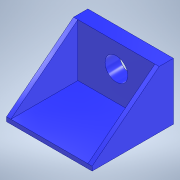
# Autodesk Inventor part: Motor Mount
Saved by Autodesk Inventor 2022 (Build 260153000, 153)
## iProperties
Created: 2022-08-10
Part Number: Motor Mount
Material: Generic
Document SubType Name: Modeling
Designer: Nick
Density: 1 g/cm^3
Appearance: Blue - Wall Paint - Glossy
Author: Nick
Autodesk Inventor part; units mm, degrees
ref_plane "YZ Plane" through (0, 0, 0) normal (1, 0, 0) x (0, 1, 0)
ref_plane "XZ Plane" through (0, 0, 0) normal (0, 1, 0) x (-1, 0, 0)
ref_plane "XY Plane" through (0, 0, 0) normal (0, 0, 1) x (1, 0, 0)
sketch "Sketch14" plane through (0, 0, 0) normal (0, 0, 1) x (1, 0, 0)
  line L0 (0, 0) -> (60, 0)
  line L1 (60, 0) -> (60, 40)
  line L2 (60, 40) -> (0, 40)
  line L3 (0, 40) -> (0, 0)
  circle A0 centre (30, 23.5) radius 8
  point P0 (60, 20)
  point P1 (30, 40)
  dimension "d94" = 16
  dimension "d95" = 60
  dimension "d96" = 40
  dimension "d104" = 23.5
  constraints: 8 end point, 2 midpoint, 2 parallel, 1 centre point, 1 horizontal, 1 perpendicular, 1 vertical alignment
  measures "d94" diameter of A0
  measures "d95" distance of L0.start L0.end
  measures "d96" distance of L2.end L0.start
  measures "d104" distance from line of L0 A0.centre
extrude "Extrusion13" add sketch "Sketch14" along normal blind 10
sketch "Sketch15" plane through (0, 0, 0) normal (0, -1, 0) x (1, 0, 0)
  line L0 (0, 0) -> (60, 0) projected
  line L1 (60, 0) -> (60, 10) projected
  line L2 (0, 10) -> (60, 10) projected
  line L3 (0, 0) -> (0, 10) projected
  line L4 (60, 0) -> (60, 10) projected
  line L5 (60, 10) -> (0, 10)
  line L6 (0, 10) -> (0, 57)
  line L7 (0, 57) -> (60, 57)
  line L8 (60, 57) -> (60, 10)
  line L9 (0, 0) -> (0, 10) projected
  dimension "d99" = 47
  constraints: 8 end point, 2 parallel, 1 collinear, 1 horizontal, 1 perpendicular
  measures "d99" distance of L7.end L1.end
extrude "Extrusion14" add sketch "Sketch15" against normal blind 3 contours L6 L7 L8 L2
sketch "Sketch16" plane through (60, 0, 0) normal (1, 0, 0) x (0, 0, -1)
  line L0 (0, 0) -> (0, 40) projected
  line L1 (0, 40) -> (-10, 40) projected
  line L2 (-10, 3) -> (-10, 40) projected
  line L3 (-57, 3) -> (-10, 3) projected
  line L4 (-57, 0) -> (-57, 3) projected
  line L5 (0, 0) -> (-57, 0) projected
  line L6 (0, 40) -> (-10, 40) projected
  line L7 (-10, 3) -> (-57, 3) projected
  line L8 (-10, 40) -> (-57, 3)
  point P0 (0, 0)
  constraints: 2 end point
extrude "Extrusion15" add sketch "Sketch16" against normal blind 3 contours L2 L3 L8
ref_plane "Work Plane3" through (30, 0, 0) normal (1, 0, 0) x (0, 0, -1)
mirror "Mirror3" about plane through (30, 0, 0) normal (1, 0, 0) of "Extrusion15"
body "Solid3"
